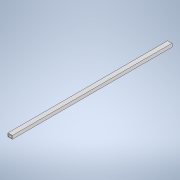
# Autodesk Inventor part: 1x0.75x0.125x36inAluminumExtrusion
Saved by Autodesk Inventor 2020.2 (Build 242310000, 310)
## iProperties
Created: 2020-01-12
Part Number: 1x0.75x0.125x36inAluminumExtrusion
Material: Generic
Document SubType Name: Modeling
Designer: robst
Density: 1 g/cm^3
Appearance: Default
Author: robst
Autodesk Inventor part; units mm, degrees
ref_plane "YZ Plane" through (0, 0, 0) normal (1, 0, 0) x (0, 1, 0)
ref_plane "XZ Plane" through (0, 0, 0) normal (0, 1, 0) x (-1, 0, 0)
ref_plane "XY Plane" through (0, 0, 0) normal (0, 0, 1) x (1, 0, 0)
sketch "Sketch1" plane through (0, 0, 0) normal (0, 0, 1) x (1, 0, 0)
  line L0 (-12.7, -9.525) -> (12.7, -9.525)
  line L1 (12.7, -9.525) -> (12.7, 9.525)
  line L2 (12.7, 9.525) -> (-12.7, 9.525)
  line L3 (-12.7, 9.525) -> (-12.7, -9.525)
  line L4 (-12.7, -9.525) -> (12.7, 9.525) construction
  line L5 (12.7, -9.525) -> (-12.7, 9.525) construction
  line L6 (-9.525, -6.35) -> (9.525, -6.35)
  line L7 (9.525, -6.35) -> (9.525, 6.35)
  line L8 (9.525, 6.35) -> (-9.525, 6.35)
  line L9 (-9.525, 6.35) -> (-9.525, -6.35)
  line L10 (-9.525, -6.35) -> (9.525, 6.35) construction
  line L11 (9.525, -6.35) -> (-9.525, 6.35) construction
  point P0 (0, 0)
  dimension "d0" = 25.4
  dimension "d1" = 19.05
  dimension "d2" = 3.175
  dimension "d3" = 3.175
  constraints: 24 end point, 5 parallel, 4 midpoint, 2 perpendicular, 1 horizontal
  measures "d0" distance of L0.start L0.end
  measures "d1" distance of L1.end L0.end
  measures "d2" distance between parallel lines of L0 L6
  measures "d3" distance between parallel lines of L3 L9
extrude "Extrusion1" add sketch "Sketch1" along normal blind 914.4
body "Solid1"
